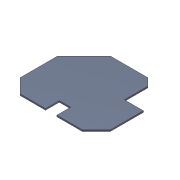
# Autodesk Inventor part: Pb_TX_bot
Saved by Autodesk Inventor 2014 SP1 (Build 180222100, 222)
## iProperties
Created: 2013-09-02
Part Number: Pb_TX_bot
Document SubType Name: Modeling
Designer: Robert Davis
Density: 11.37 g/cm^3
Material: Lead
Mass: 118.558 g
Surface Area: 137.996 cm^2
Volume: 10.4273 cm^3
Appearance: Lead
Author: Robert Davis
Autodesk Inventor part; units mm, degrees
ref_plane "YZ Plane" through (0, 0, 0) normal (1, 0, 0) x (0, 1, 0)
ref_plane "XZ Plane" through (0, 0, 0) normal (0, 1, 0) x (-1, 0, 0)
ref_plane "XY Plane" through (0, 0, 0) normal (0, 0, 1) x (1, 0, 0)
sketch "Sketch1" plane through (0, 0, 0) normal (0, 0, 1) x (1, 0, 0)
  line L0 (0, 0) -> (0, 24.8008)
  line L1 (0, 0) -> (23.5103, 0)
  line L2 (-19.7, 47.5) -> (19.7, 47.5)
  line L3 (47.5, 19.7) -> (47.5, -19.7)
  line L4 (19.7, -47.5) -> (-19.7, -47.5)
  line L5 (-47.5, -19.7) -> (-47.5, 19.7)
  line L6 (19.7, 47.5) -> (47.5, 19.7)
  line L7 (47.5, -19.7) -> (19.7, -47.5)
  line L8 (-19.7, -47.5) -> (-47.5, -19.7)
  line L9 (-47.5, 19.7) -> (-19.7, 47.5)
  point P0 (-47.5, 47.5)
  point P1 (47.5, -47.5)
  point P2 (47.5, 47.5)
  point P3 (-47.5, -47.5)
  dimension "d9" = 27.8
  dimension "d10" = 27.8
  dimension "d11" = 27.8
  dimension "d12" = 27.8
  dimension "d13" = 27.8
  dimension "d14" = 27.8
  dimension "d15" = 27.8
  dimension "d16" = 27.8
  dimension "d17" = 95
  dimension "d18" = 95
  constraints: 20 end point, 8 point on line, 2 horizontal, 2 vertical, 1 coincident, 3 other
  measures "d9" distance of L2.end point (47.5, 47.5)
  measures "d10" distance of L3.start point (47.5, 47.5)
  measures "d11" distance of L3.end point (47.5, -47.5)
  measures "d12" distance of L4.start point (47.5, -47.5)
  measures "d13" distance of L4.end point (-47.5, -47.5)
  measures "d14" distance of L5.start point (-47.5, -47.5)
  measures "d15" distance of L5.end point (-47.5, 47.5)
  measures "d16" distance of L2.start point (-47.5, 47.5)
  measures "d17" distance between parallel lines of L4 L2
  measures "d18" distance between parallel lines of L3 L5
extrude "Extrusion1" add sketch "Sketch1" along normal mid plane 1.5748
sketch "Sketch4" plane through (0, 0, 0.7874) normal (0, 0, 1) x (1, 0, 0)
  line L0 (19.7, -47.5) -> (-19.7, -47.5) projected
  line L1 (-35, -47.5) -> (35, -47.5)
  line L2 (35, -47.5) -> (35, -34.5)
  line L3 (35, -34.5) -> (-35, -34.5)
  line L4 (-35, -34.5) -> (-35, -47.5)
  point P0 (12, -47.5)
  point P1 (0, 0)
  point P2 (0, -34.5)
  dimension "d24" = 13
  dimension "d25" = 70
  constraints: 8 end point, 2 horizontal, 2 vertical, 1 collinear, 1 midpoint, 1 vertical alignment
  measures "d24" distance of L1.end L2.end
  measures "d25" distance of L2.end L3.end
extrude "Extrusion4" cut sketch "Sketch4" against normal through all
sketch "Sketch5" plane through (0, 0, 0.7874) normal (0, 0, 1) x (1, 0, 0)
  line L0 (-6, -47.5) -> (6, -47.5)
  line L1 (6, -47.5) -> (6, -20)
  line L2 (6, -20) -> (-6, -20)
  line L3 (-6, -20) -> (-6, -47.5)
  line L4 (0, 0) -> (0, -10.8647)
  dimension "d29" = 12
  dimension "d30" = 27.5
  dimension "d45" = 20
  constraints: 10 end point, 2 vertical, 1 coincident, 1 horizontal, 1 other
  measures "d29" distance of L1.end L2.end
  measures "d30" distance of L0.end L1.end
  measures "d45" distance from line of point (0, 0) L2
extrude "Extrusion5" cut sketch "Sketch5" against normal through all
sketch "Sketch7" plane through (0, 0, -0.7874) normal (0, 0, -1) x (-1, 0, 0)
  line L0 (-47.5, -19.7) -> (-47.5, 19.7) projected
  line L1 (-47.5, 40) -> (-27.5, 40)
  line L2 (-27.5, 40) -> (-27.5, 15)
  line L3 (-27.5, 15) -> (-47.5, 15)
  line L4 (-47.5, 15) -> (-47.5, 40)
  point P0 (0, 0)
  point P1 (-27.5, 27.5)
  point P2 (-27.5, 27.5)
  dimension "d37" = 25
  dimension "d38" = 20
  dimension "d46" = 15
  constraints: 8 end point, 2 horizontal, 1 coincident, 1 collinear, 1 midpoint, 1 vertical
  measures "d37" distance of L3.end L1.start
  measures "d38" distance of L1.start L1.end
  measures "d46" distance from line of point (0, 0) L3
extrude "Extrusion7" cut sketch "Sketch7" against normal through all
equation "\"d10\" = d9"
equation "\"d11\" = d9"
equation "\"d12\" = d11"
equation "\"d13\" = d9"
equation "\"d14\" = d13"
equation "\"d15\" = d9"
equation "\"d16\" = d15"
body "Solid1"
